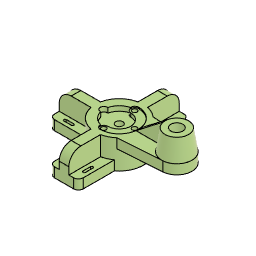
Exercise-15 v1 (Autodesk Fusion 360 design; units mm, degrees)
Autodesk Fusion 360 part; units mm, degrees
sketch "Sketch1" plane through (0, 0, 0) normal (0, 0, 1) x (1, 0, 0)
  circle A0 centre (0, 0) radius 500
  line L0 (1150, -300) -> (-1150, -300)
  line L1 (-1150, -300) -> (-1150, 300)
  line L2 (-1150, 300) -> (1150, 300)
  line L3 (1150, 300) -> (1150, -300)
  line L4 (300, -1150) -> (-300, -1150)
  line L5 (-300, -1150) -> (-300, 1150)
  line L6 (-300, 1150) -> (300, 1150)
  line L7 (300, 1150) -> (300, -1150)
  line L8 (1150, -100) -> (-1150, -100)
  line L9 (-1150, -100) -> (-1150, 100)
  line L10 (-1150, 100) -> (1150, 100)
  line L11 (1150, 100) -> (1150, -100)
  line L12 (100, -1150) -> (-100, -1150)
  line L13 (-100, -1150) -> (-100, 1150)
  line L14 (-100, 1150) -> (100, 1150)
  line L15 (100, 1150) -> (100, -1150)
  line L16 (-930, -225) -> (-770, -225)
  arc A1 (-770, -225) -> (-770, -175) centre (-770, -200) ccw
  line L17 (-770, -175) -> (-930, -175)
  arc A2 (-930, -175) -> (-930, -225) centre (-930, -200) ccw
  line L18 (-930, -200) -> (-770, -200) construction
  line L19 (-1150, 0) -> (-817.5132, 0) construction
  line L20 (-770, 175) -> (-930, 175)
  arc A3 (-770, 175) -> (-770, 225) centre (-770, 200) ccw
  line L21 (-930, 225) -> (-770, 225)
  arc A4 (-930, 225) -> (-930, 175) centre (-930, 200) ccw
  line L22 (175, -770) -> (175, -930)
  line L23 (225, -930) -> (225, -770)
  arc A5 (225, -770) -> (175, -770) centre (200, -770) ccw
  arc A6 (175, -930) -> (225, -930) centre (200, -930) ccw
  line L24 (-225, -930) -> (-225, -770)
  arc A7 (-225, -930) -> (-175, -930) centre (-200, -930) ccw
  line L25 (-175, -770) -> (-175, -930)
  arc A8 (-175, -770) -> (-225, -770) centre (-200, -770) ccw
  line L26 (-175, 770) -> (-175, 930)
  line L27 (-225, 930) -> (-225, 770)
  arc A9 (-225, 770) -> (-175, 770) centre (-200, 770) ccw
  arc A10 (-175, 930) -> (-225, 930) centre (-200, 930) ccw
  line L28 (225, 930) -> (225, 770)
  arc A11 (225, 930) -> (175, 930) centre (200, 930) ccw
  line L29 (175, 770) -> (175, 930)
  arc A12 (175, 770) -> (225, 770) centre (200, 770) ccw
  dimension "d2" = 2300
  dimension "d3" = 600
  dimension "d4" = 600
  dimension "d5" = 2300
  dimension "d6" = 2300
  dimension "d7" = 200
  dimension "d8" = 200
  dimension "d9" = 2300
  dimension "d10" = 160
  dimension "d11" = 50
  dimension "d12" = 220
  dimension "d13" = 100
  dimension "d15" = 360
  constraint coincident A0.centre origin
  constraint horizontal L0
  constraint perpendicular L0 L1
  constraint parallel L0 L2
  constraint parallel L1 L3
  constraint horizontal L4
  constraint perpendicular L4 L5
  constraint parallel L4 L6
  constraint parallel L5 L7
  constraint horizontal L8
  constraint perpendicular L8 L9
  constraint parallel L8 L10
  constraint parallel L9 L11
  constraint horizontal L12
  constraint perpendicular L12 L13
  constraint parallel L12 L14
  constraint parallel L13 L15
  constraint tangent L16 A1
  constraint tangent A1 L17
  constraint parallel L16 L17
  constraint tangent L17 A2
  constraint tangent L16 A2
  constraint horizontal L18
  constraint midpoint L9 L19.start
  constraint perpendicular L9 L19
  constraint symmetric L16.start L19 L21.start
  constraint symmetric L16.end L19 A3.end
  constraint symmetric A1.end L19 L20.start
  constraint symmetric L17.end L19 L20.end
  constraint symmetric A1 L19 A3
  constraint symmetric A2 L19 A4
  measures "d2" distance of L1.end L2.end
  measures "d3" distance of L0.end L1.end
  measures "d4" distance of L5.end L6.end
  measures "d5" distance of L4.end L5.end
  measures "d6" distance of L9.end L10.end L5.end
  measures "d7" distance of L8.end L9.end L5.end
  measures "d8" distance of L13.end L14.end L5.end
  measures "d9" distance of L12.end L13.end L5.end
  measures "d10" distance of A2.centre A1.centre
  measures "d11" diameter of A1
  measures "d12" distance of L1 A2.centre
  measures "d13" distance of L0 A2.centre
extrude "Extrude1" add sketch "Sketch1" along normal blind 600 contours A0 L7 L8 L10 | A0 L2 L7 L10 | A0 L0 L7 L8 | A0 L2 L7 | L2 L7 L10 L15 | L7 L8 L10 L15 | A0 L0 L7 | L0 L7 L8 L15 | A0 L2 L7 L15 | L8 L10 L13 L15 | L2 L10 L13 L15 | A0 L0 L7 L15 | L0 L8 L13 L15 | A0 L2 L13 L15 | A0 L6 L13 L14 L15 | L5 L8 L10 L13 | L2 L5 L10 L13 | A0 L4 L12 L13 L15 | A0 L0 L13 L15 | L0 L5 L8 L13 | A0 L2 L5 L13 | A0 L2 L5 L10 | A0 L5 L8 L10 | A0 L0 L5 L13 | A0 L0 L5 L8 | A0 L2 L5 | A0 L1 L8 L9 L10 | A0 L0 L5 makes body 1
extrude "Extrude2" add sketch "Sketch1" along normal blind 200 contours A0 L6 L7 L15 | A0 L4 L7 L15 | A0 L5 L6 L13 | A0 L4 L5 L13 | A0 L1 L2 L10 | A0 L0 L1 L8 bodies 1
sketch "Sketch2" plane through (0, 0, 600) normal (0, 0, 1) x (-1, 0, 0)
  arc A0 (100, -489.8979) -> (489.8979, -100) centre (0, 0) ccw
  line L0 (489.8979, -100) -> (1150, -100)
  line L1 (1150, -100) -> (1150, 100)
  line L2 (1150, 100) -> (489.8979, 100)
  arc A1 (489.8979, 100) -> (100, 489.8979) centre (0, 0) ccw
  line L3 (100, 489.8979) -> (100, 1150)
  line L4 (100, 1150) -> (-100, 1150)
  line L5 (-100, 1150) -> (-100, 489.8979)
  arc A2 (-100, 489.8979) -> (-100, -489.8979) centre (0, 0) ccw
  line L6 (-100, -489.8979) -> (-100, -1150)
  line L7 (-100, -1150) -> (100, -1150)
  line L8 (100, -1150) -> (100, -489.8979)
  circle A3 centre (0, 0) radius 320
  circle A4 centre (0, 0) radius 400
  circle A5 centre (0, 0) radius 240
  circle A6 centre (0, 0) radius 75
  circle A7 centre (320, 0) radius 75
  circle A8 centre (0, -320) radius 80
  circle A9 centre (0, 320) radius 80
  circle A10 centre (-1200, 0) radius 315
  circle A11 centre (-1200, 0) radius 125
  line L9 (-28.3333, -398.9953) -> (-1222.3125, -314.2088)
  line L10 (-28.3333, 398.9953) -> (-1222.3125, 314.2088)
  circle A12 centre (0, -320) radius 50
  circle A13 centre (0, 320) radius 50
  circle A14 centre (-320, 0) radius 50
  line L11 (0, 0) -> (-75, 0) construction
  dimension "d20" = 640
  dimension "d21" = 800
  dimension "d22" = 480
  dimension "d23" = 150
  dimension "d24" = 150
  dimension "d25" = 160
  dimension "d27" = 160
  dimension "d28" = 630
  dimension "d29" = 250
  dimension "d30" = 2350
  dimension "d34" = 100
  dimension "d35" = 100
  dimension "d36" = 100
  constraint concentric A0 A3
  constraint concentric A0 A4
  constraint concentric A0 A5
  constraint concentric A5 A6
  constraint coincident A3 A7.centre
  constraint coincident A3 A8.centre
  constraint coincident A3 A9.centre
  constraint concentric A10 A11
  constraint coincident A4 L9.start
  constraint coincident A10 L9.end
  constraint tangent A10 L9
  constraint tangent A4 L9
  constraint coincident A0.centre A1.centre
  constraint horizontal L11
  constraint symmetric L9.start L10.start L11
  constraint symmetric L9.end L10.end L11
  constraint concentric A8 A12
  constraint concentric A9 A13
  constraint coincident A6 L11.end
  measures "d20" diameter of A3
  measures "d21" diameter of A4
  measures "d22" diameter of A5
  measures "d23" diameter of A6
  measures "d24" diameter of A7
  measures "d25" diameter of A8
  measures "d27" diameter of A9
  measures "d28" diameter of A10
  measures "d29" diameter of A11
  measures "d30" distance of L1 A10.centre
  measures "d34" diameter of A12
  measures "d35" diameter of A13
  measures "d36" diameter of A14
extrude "Extrude3" add sketch "Sketch2" against normal blind 200 contours A2 A10 L9 L10 | A10 | A11 bodies 1
extrude "Extrude4" cut sketch "Sketch2" against normal through all contours A6 bodies 1
extrude "Extrude5" cut sketch "Sketch2" against normal blind 100 contours A5 | A3 A5 A7 A8 A9 | A3 A7 | A3 A7 bodies 1
extrude "Extrude6" cut sketch "Sketch2" against normal blind 200 contours A3 A14 | A3 A14 | A3 A12 | A3 A12 | A3 A13 | A3 A13 bodies 1
extrude "Extrude7" cut sketch "Sketch2" against normal blind 25 contours A3 A4 A8 A9 A14 | A3 A8 A12 | A3 A9 A13 | A3 A8 A12 | A3 A5 A8 A9 A14 | A3 A9 A13 bodies 1
sketch "Sketch3" plane through (0, 0, 400) normal (0, 0, -1) x (1, 0, 0)
  arc A0 (1222.3125, -314.2088) -> (1222.3125, 314.2088) centre (1200, 0) ccw
  line L0 (1222.3125, 314.2088) -> (327.5798, 377.7453)
  arc A1 (327.5798, -377.7453) -> (327.5798, 377.7453) centre (0, 0) ccw
  line L1 (327.5798, -377.7453) -> (1222.3125, -314.2088)
  circle A2 centre (1200, 0) radius 225
  dimension "d43" = 450
  constraint concentric A0 A2
  measures "d43" diameter of A2
sketch "Sketch4" plane through (0, 0, 0) normal (0, 1, 0) x (1, 0, 0)
ref_plane "WorkPlane1" through (182.5, 0, 1030) normal (0, 0, 1) x (1, 0, 0)
sketch "Sketch5" plane through (0, 0, 1030) normal (0, 0, 1) x (1, 0, 0)
  circle A0 centre (1200, 0) radius 125
  point P0 (1200, 0)
  dimension "d46" = 250
  constraint coincident P0 A0.centre
  measures "d46" diameter of A0
loft "Loft1" add profiles "Sketch3", "Sketch5" section 1 contours A2 section 2 separate body makes body 2
sketch "Sketch6" plane through (0, 0, 0) normal (0, 1, 0) x (1, 0, 0)
  line L0 (1325, -1030) -> (1075, -1030)
  line L1 (975, -400) -> (1425, -400)
  line L2 (1325, -1030) -> (1425, -400)
  line L3 (1075, -1030) -> (975, -400)
  line L4 (-1150, -600) -> (-489.8979, -600)
  line L5 (-489.8979, -600) -> (-100, -600)
  line L6 (-100, -600) -> (100, -600)
  line L7 (100, -600) -> (327.5798, -600)
  line L8 (327.5798, -600) -> (1222.3125, -600)
  line L9 (1222.3125, -600) -> (1515, -600)
  line L10 (1222.3125, -400) -> (500, -400)
  line L11 (1515, -400) -> (1222.3125, -400)
  line L12 (-400, 0) -> (-300, 0)
  line L13 (300, 0) -> (500, 0)
  line L14 (-400, 0) -> (-1150, 0)
  line L15 (-1150, 0) -> (-1150, -200)
  line L16 (300, 0) -> (-300, 0)
  line L17 (-1150, -200) -> (-1150, -600)
  line L18 (1515, -600) -> (1515, -400)
  line L19 (500, 0) -> (500, -400)
  line L20 (1515, -600) -> (1446.746, -1030)
  line L21 (1446.746, -1030) -> (1325, -1030)
  line L22 (1200, -1030) -> (1200, -772.2926) construction
  line L23 (885, -600) -> (953.254, -1030)
  line L24 (953.254, -1030) -> (1075, -1030)
  arc A0 through (0, -600, -400) (400, -600, 0) (0, -600, 400)
  line L25 (953.254, -1030) -> (400, -600)
  constraint coincident L9.end L18.start
  constraint parallel L2 L20
  constraint coincident L0.start L2.start
  constraint parallel L0 L21
  constraint midpoint L0 L22.start
  constraint perpendicular L0 L22
  constraint symmetric L9.end L22 L23.start
  constraint symmetric L20.end L22 L23.end
  constraint symmetric L0.start L22 L0.end
revolve "Revolve1" add sketch "Sketch6" angle 360 about axis through (1200, 0, 400) along (0, 0, 1) separate body contours L2 L9 L20 L21 makes body 3
extrude "Extrude8" add sketch "Sketch6" along normal mid plane 100 separate body contours L8 L23 L25 makes body 4
combine "Combine1" operation add target body 3 tool bodies 4 1
combine "Combine2" operation cut target body 3 tool bodies 2
fillet "Fillet1" radius 250 3 edges at (0, -1150, 600) (-1150, 0, 600) (0, 1150, 600) on bodies 3
fillet "Fillet2" radius 100 6 edges at (-1150, -300, 100) (-300, -1150, 100) (300, -1150, 100) (300, 1150, 100) (-1150, 300, 100) (-300, 1150, 100) on bodies 3
